Autodesk Fusion 360 part; units mm, degrees
(part 2 of 2)
sketch "Sketch6" plane through (0, 0, 2) normal (0, 0, 1) x (-1, 0, 0)
  spline S0 degree 3 poles (34.098, 26.8331) (34.098, 26.5964) (33.9796, 26.4781) (33.743, 26.4781) knots 0 0 0 0 1 1 1 1
  spline S1 degree 3 poles (33.743, 26.4781) (33.6225, 26.4812) (33.5343, 26.5113) (33.4772, 26.5694) knots 0 0 0 0 1 1 1 1
  spline S2 degree 3 poles (33.4772, 26.5694) (33.4206, 26.6276) (33.1512, 26.8965) (32.6695, 27.375) knots 0 0 0 0 1 1 1 1
  spline S3 degree 3 poles (32.6695, 27.375) (32.1935, 26.8991) (31.9257, 26.6307) (31.866, 26.5694) knots 0 0 0 0 1 1 1 1
  spline S4 degree 3 poles (31.866, 26.5694) (31.8068, 26.5087) (31.7181, 26.4781) (31.6003, 26.4781) knots 0 0 0 0 1 1 1 1
  spline S5 degree 3 poles (31.6003, 26.4781) (31.3636, 26.4796) (31.2447, 26.598) (31.2431, 26.8331) knots 0 0 0 0 1 1 1 1
  line L0 (31.2431, 26.8331) -> (31.2411, 28.9738)
  spline S6 degree 3 poles (31.2411, 28.9738) (31.2411, 29.2105) (31.3615, 29.3309) (31.6023, 29.335) knots 0 0 0 0 1 1 1 1
  spline S7 degree 3 poles (31.6023, 29.335) (31.838, 29.3335) (31.9569, 29.2136) (31.9594, 28.9738) knots 0 0 0 0 1 1 1 1
  line L1 (31.9594, 28.9738) -> (31.9594, 27.7135)
  spline S8 degree 3 poles (31.9594, 27.7135) (32.1993, 27.9585) (32.3487, 28.1116) (32.4079, 28.1723) knots 0 0 0 0 1 1 1 1
  spline S9 degree 3 poles (32.4079, 28.1723) (32.4661, 28.232) (32.5543, 28.2616) (32.6716, 28.2616) knots 0 0 0 0 1 1 1 1
  spline S10 degree 3 poles (32.6716, 28.2616) (32.7868, 28.2616) (32.8746, 28.2315) (32.9353, 28.1702) knots 0 0 0 0 1 1 1 1
  spline S11 degree 3 poles (32.9353, 28.1702) (32.9965, 28.108) (33.146, 27.9579) (33.3838, 27.7197) knots 0 0 0 0 1 1 1 1
  line L2 (33.3838, 27.7197) -> (33.3838, 28.9738)
  spline S12 degree 3 poles (33.3838, 28.9738) (33.3853, 29.2094) (33.5042, 29.3283) (33.7409, 29.3309) knots 0 0 0 0 1 1 1 1
  spline S13 degree 3 poles (33.7409, 29.3309) (33.9807, 29.3319) (34.0996, 29.2136) (34.098, 28.9738) knots 0 0 0 0 1 1 1 1
  line L3 (34.098, 28.9738) -> (34.098, 26.8331)
  spline S14 degree 3 poles (1.992, 26.8352) (1.992, 26.6001) (1.8731, 26.4812) (1.6349, 26.4781) knots 0 0 0 0 1 1 1 1
  line L4 (1.6349, 26.4781) -> (0.3871, 26.4781)
  spline S15 degree 3 poles (0.3871, 26.4781) (0.1504, 26.4781) (-0.0578, 26.5674) (-0.2379, 26.7459) knots 0 0 0 0 1 1 1 1
  spline S16 degree 3 poles (-0.2379, 26.7459) (-0.4191, 26.9245) (-0.5083, 27.1332) (-0.5057, 27.3709) knots 0 0 0 0 1 1 1 1
  spline S17 degree 3 poles (-0.5057, 27.3709) (-0.5026, 27.6091) (-0.4414, 27.7856) (-0.3209, 27.9003) knots 0 0 0 0 1 1 1 1
  spline S18 degree 3 poles (-0.3209, 27.9003) (-0.4466, 28.0239) (-0.5083, 28.2029) (-0.5057, 28.4381) knots 0 0 0 0 1 1 1 1
  spline S19 degree 3 poles (-0.5057, 28.4381) (-0.5042, 28.6737) (-0.4144, 28.8814) (-0.2358, 29.061) knots 0 0 0 0 1 1 1 1
  spline S20 degree 3 poles (-0.2358, 29.061) (-0.0573, 29.2411) (0.1431, 29.3309) (0.3642, 29.3309) knots 0 0 0 0 1 1 1 1
  line L5 (0.3642, 29.3309) -> (1.639, 29.3309)
  spline S21 degree 3 poles (1.639, 29.3309) (1.8747, 29.3335) (1.992, 29.2146) (1.992, 28.9738) knots 0 0 0 0 1 1 1 1
  line L6 (1.992, 28.9738) -> (1.992, 26.8352)
  spline S22 degree 3 poles (-8.0953, 26.5611) (-8.1587, 26.5004) (-8.249, 26.4698) (-8.3653, 26.4698) knots 0 0 0 0 1 1 1 1
  spline S23 degree 3 poles (-8.3653, 26.4698) (-8.4841, 26.4698) (-8.5734, 26.4999) (-8.6331, 26.5591) knots 0 0 0 0 1 1 1 1
  spline S24 degree 3 poles (-8.6331, 26.5591) (-8.6923, 26.6172) (-8.904, 26.8658) (-9.2684, 27.3044) knots 0 0 0 0 1 1 1 1
  spline S25 degree 3 poles (-9.2684, 27.3044) (-9.6364, 26.8575) (-9.8503, 26.6058) (-9.91, 26.5487) knots 0 0 0 0 1 1 1 1
  spline S26 degree 3 poles (-9.91, 26.5487) (-9.9707, 26.4905) (-10.0605, 26.4615) (-10.1799, 26.4615) knots 0 0 0 0 1 1 1 1
  spline S27 degree 3 poles (-10.1799, 26.4615) (-10.2962, 26.4615) (-10.3855, 26.4921) (-10.4477, 26.5528) knots 0 0 0 0 1 1 1 1
  spline S28 degree 3 poles (-10.4477, 26.5528) (-10.51, 26.6125) (-10.5396, 26.7023) (-10.537, 26.8227) knots 0 0 0 0 1 1 1 1
  spline S29 degree 3 poles (-10.537, 26.8227) (-10.537, 26.9489) (-10.4737, 27.0667) (-10.3481, 27.1757) knots 0 0 0 0 1 1 1 1
  line L7 (-10.3481, 27.1757) -> (-9.7397, 27.892)
  line L8 (-9.7397, 27.892) -> (-10.3481, 28.6021)
  spline S30 degree 3 poles (-10.3481, 28.6021) (-10.482, 28.7282) (-10.5443, 28.8492) (-10.5349, 28.9655) knots 0 0 0 0 1 1 1 1
  spline S31 degree 3 poles (-10.5349, 28.9655) (-10.5401, 29.0859) (-10.5105, 29.1762) (-10.4457, 29.2354) knots 0 0 0 0 1 1 1 1
  spline S32 degree 3 poles (-10.4457, 29.2354) (-10.3803, 29.2951) (-10.2905, 29.3241) (-10.1758, 29.3226) knots 0 0 0 0 1 1 1 1
  spline S33 degree 3 poles (-10.1758, 29.3226) (-10.0522, 29.3241) (-9.9603, 29.293) (-9.8996, 29.2291) knots 0 0 0 0 1 1 1 1
  spline S34 degree 3 poles (-9.8996, 29.2291) (-9.8384, 29.1658) (-9.6307, 28.9193) (-9.2767, 28.49) knots 0 0 0 0 1 1 1 1
  spline S35 degree 3 poles (-9.2767, 28.49) (-8.9155, 28.9276) (-8.7042, 29.1772) (-8.6435, 29.2395) knots 0 0 0 0 1 1 1 1
  spline S36 degree 3 poles (-8.6435, 29.2395) (-8.5822, 29.3018) (-8.4903, 29.3319) (-8.3673, 29.3309) knots 0 0 0 0 1 1 1 1
  spline S37 degree 3 poles (-8.3673, 29.3309) (-8.2521, 29.3335) (-8.1623, 29.3054) (-8.0974, 29.2457) knots 0 0 0 0 1 1 1 1
  spline S38 degree 3 poles (-8.0974, 29.2457) (-8.032, 29.185) (-8.0029, 29.0942) (-8.0102, 28.9738) knots 0 0 0 0 1 1 1 1
  spline S39 degree 3 poles (-8.0102, 28.9738) (-7.9988, 28.8575) (-8.0606, 28.7371) (-8.195, 28.6125) knots 0 0 0 0 1 1 1 1
  line L9 (-8.195, 28.6125) -> (-8.8303, 27.9024)
  line L10 (-8.8303, 27.9024) -> (-8.1971, 27.1861)
  spline S40 degree 3 poles (-8.1971, 27.1861) (-8.0709, 27.0755) (-8.0081, 26.9572) (-8.0081, 26.8311) knots 0 0 0 0 1 1 1 1
  spline S41 degree 3 poles (-8.0081, 26.8311) (-8.004, 26.7106) (-8.033, 26.6208) (-8.0953, 26.5611) knots 0 0 0 0 1 1 1 1
  spline S42 degree 3 poles (13.2978, 6.9999) (13.8352, 7.003) (14.106, 6.7343) (14.1081, 6.1938) knots 0 0 0 0 1 1 1 1
  spline S43 degree 3 poles (14.1081, 6.1938) (14.1029, 5.6543) (13.8342, 5.3794) (13.3019, 5.3711) knots 0 0 0 0 1 1 1 1
  line L11 (13.3019, 5.3711) -> (11.6648, 5.3711)
  spline S44 degree 3 poles (11.6648, 5.3711) (11.1222, 5.3773) (10.8463, 5.6481) (10.838, 6.1855) knots 0 0 0 0 1 1 1 1
  spline S45 degree 3 poles (10.838, 6.1855) (10.8494, 6.7292) (11.1233, 6.9999) (11.6607, 6.9999) knots 0 0 0 0 1 1 1 1
  line L12 (11.6607, 6.9999) -> (13.2978, 6.9999)
  spline S46 degree 3 poles (24.2533, 2.9237) (23.7158, 2.9268) (23.4451, 3.1986) (23.4388, 3.7381) knots 0 0 0 0 1 1 1 1
  spline S47 degree 3 poles (23.4388, 3.7381) (23.4388, 4.2818) (23.7014, 4.5546) (24.2243, 4.5567) knots 0 0 0 0 1 1 1 1
  line L13 (24.2243, 4.5567) -> (26.7007, 4.5525)
  spline S48 degree 3 poles (26.7007, 4.5525) (27.2495, 4.5587) (27.5265, 4.6962) (27.5316, 4.966) knots 0 0 0 0 1 1 1 1
  spline S49 degree 3 poles (27.5316, 4.966) (27.5234, 5.2254) (27.2453, 5.3535) (26.6965, 5.3504) knots 0 0 0 0 1 1 1 1
  line L14 (26.6965, 5.3504) -> (25.8945, 5.3504)
  spline S50 degree 3 poles (25.8945, 5.3504) (24.2605, 5.3566) (23.4388, 6.0439) (23.4306, 7.4134) knots 0 0 0 0 1 1 1 1
  spline S51 degree 3 poles (23.4306, 7.4134) (23.4306, 8.7445) (24.2512, 9.4143) (25.8904, 9.4225) knots 0 0 0 0 1 1 1 1
  line L15 (25.8904, 9.4225) -> (28.3378, 9.4225)
  spline S52 degree 3 poles (28.3378, 9.4225) (28.8814, 9.4205) (29.1512, 9.1538) (29.1481, 8.6247) knots 0 0 0 0 1 1 1 1
  spline S53 degree 3 poles (29.1481, 8.6247) (29.146, 8.0851) (28.8783, 7.8175) (28.346, 7.8226) knots 0 0 0 0 1 1 1 1
  line L16 (28.346, 7.8226) -> (25.8904, 7.8102)
  spline S54 degree 3 poles (25.8904, 7.8102) (25.3447, 7.8082) (25.0718, 7.6686) (25.0718, 7.3927) knots 0 0 0 0 1 1 1 1
  spline S55 degree 3 poles (25.0718, 7.3927) (25.0718, 7.1147) (25.3478, 6.9772) (25.8986, 6.9793) knots 0 0 0 0 1 1 1 1
  line L17 (25.8986, 6.9793) -> (26.7007, 6.9793)
  spline S56 degree 3 poles (26.7007, 6.9793) (28.3326, 6.9772) (29.1481, 6.3054) (29.1481, 4.966) knots 0 0 0 0 1 1 1 1
  spline S57 degree 3 poles (29.1481, 4.966) (29.1594, 3.6079) (28.344, 2.9268) (26.7007, 2.9237) knots 0 0 0 0 1 1 1 1
  line L18 (26.7007, 2.9237) -> (24.2533, 2.9237)
  spline S58 degree 3 poles (16.1297, 3.7381) (16.1276, 3.2007) (15.8558, 2.9268) (15.3153, 2.9154) knots 0 0 0 0 1 1 1 1
  line L19 (15.3153, 2.9154) -> (11.1977, 2.9237)
  spline S59 degree 3 poles (11.1977, 2.9237) (10.6912, 2.932) (10.436, 3.1955) (10.4329, 3.7133) knots 0 0 0 0 1 1 1 1
  spline S60 degree 3 poles (10.4329, 3.7133) (10.4329, 4.2673) (10.7078, 4.5484) (11.2556, 4.5567) knots 0 0 0 0 1 1 1 1
  line L20 (11.2556, 4.5567) -> (14.4967, 4.5567)
  line L21 (14.4967, 4.5567) -> (14.4967, 7.7978)
  line L22 (14.4967, 7.7978) -> (11.2638, 7.7978)
  spline S61 degree 3 poles (11.2638, 7.7978) (10.716, 7.8009) (10.4411, 8.0748) (10.4411, 8.6205) knots 0 0 0 0 1 1 1 1
  spline S62 degree 3 poles (10.4411, 8.6205) (10.4442, 9.1559) (10.7129, 9.4256) (11.2473, 9.4308) knots 0 0 0 0 1 1 1 1
  line L23 (11.2473, 9.4308) -> (15.3153, 9.4308)
  spline S63 degree 3 poles (15.3153, 9.4308) (15.8558, 9.4308) (16.1276, 9.1683) (16.1297, 8.6412) knots 0 0 0 0 1 1 1 1
  line L24 (16.1297, 8.6412) -> (16.1297, 3.7381)
  spline S64 degree 3 poles (-1.5825, 26.6629) (-1.8109, 26.5399) (-2.046, 26.4781) (-2.2884, 26.4781) knots 0 0 0 0 1 1 1 1
  spline S65 degree 3 poles (-2.2884, 26.4781) (-2.5277, 26.4781) (-2.7608, 26.5399) (-2.9881, 26.6629) knots 0 0 0 0 1 1 1 1
  spline S66 degree 3 poles (-2.9881, 26.6629) (-3.2165, 26.7864) (-3.3951, 26.9629) (-3.5238, 27.1923) knots 0 0 0 0 1 1 1 1
  spline S67 degree 3 poles (-3.5238, 27.1923) (-3.6536, 27.4207) (-3.719, 27.659) (-3.719, 27.9066) knots 0 0 0 0 1 1 1 1
  spline S68 degree 3 poles (-3.719, 27.9066) (-3.719, 28.1547) (-3.6557, 28.3919) (-3.53, 28.6187) knots 0 0 0 0 1 1 1 1
  spline S69 degree 3 poles (-3.53, 28.6187) (-3.4055, 28.8445) (-3.229, 29.0205) (-3.0006, 29.1461) knots 0 0 0 0 1 1 1 1
  spline S70 degree 3 poles (-3.0006, 29.1461) (-2.7732, 29.2722) (-2.536, 29.335) (-2.2884, 29.335) knots 0 0 0 0 1 1 1 1
  spline S71 degree 3 poles (-2.2884, 29.335) (-2.0419, 29.335) (-1.8047, 29.2722) (-1.5763, 29.1461) knots 0 0 0 0 1 1 1 1
  spline S72 degree 3 poles (-1.5763, 29.1461) (-1.3489, 29.0205) (-1.1724, 28.8445) (-1.0468, 28.6187) knots 0 0 0 0 1 1 1 1
  spline S73 degree 3 poles (-1.0468, 28.6187) (-0.9223, 28.3919) (-0.86, 28.1547) (-0.86, 27.9066) knots 0 0 0 0 1 1 1 1
  spline S74 degree 3 poles (-0.86, 27.9066) (-0.86, 27.659) (-0.9233, 27.4207) (-1.051, 27.1923) knots 0 0 0 0 1 1 1 1
  spline S75 degree 3 poles (-1.051, 27.1923) (-1.1782, 26.9629) (-1.3552, 26.7864) (-1.5825, 26.6629) knots 0 0 0 0 1 1 1 1
  spline S76 degree 3 poles (9.664, 28.2658) (9.8996, 28.2673) (10.018, 28.1495) (10.019, 27.9128) knots 0 0 0 0 1 1 1 1
  spline S77 degree 3 poles (10.019, 27.9128) (10.0164, 27.6751) (9.8986, 27.5536) (9.666, 27.5494) knots 0 0 0 0 1 1 1 1
  line L25 (9.666, 27.5494) -> (8.9476, 27.5494)
  spline S78 degree 3 poles (8.9476, 27.5494) (8.7099, 27.5526) (8.5895, 27.6719) (8.5864, 27.9086) knots 0 0 0 0 1 1 1 1
  spline S79 degree 3 poles (8.5864, 27.9086) (8.5905, 28.1469) (8.7104, 28.2658) (8.9456, 28.2658) knots 0 0 0 0 1 1 1 1
  line L26 (8.9456, 28.2658) -> (9.664, 28.2658)
  spline S80 degree 3 poles (21.9665, 26.8311) (21.9655, 26.5985) (21.8461, 26.4812) (21.6094, 26.4781) knots 0 0 0 0 1 1 1 1
  line L27 (21.6094, 26.4781) -> (20.3574, 26.4781)
  spline S81 degree 3 poles (20.3574, 26.4781) (20.1238, 26.4781) (19.9172, 26.5684) (19.7387, 26.748) knots 0 0 0 0 1 1 1 1
  spline S82 degree 3 poles (19.7387, 26.748) (19.5591, 26.9281) (19.4698, 27.1342) (19.4708, 27.3667) knots 0 0 0 0 1 1 1 1
  spline S83 degree 3 poles (19.4708, 27.3667) (19.4708, 27.6133) (19.516, 27.8214) (19.6058, 27.9917) knots 0 0 0 0 1 1 1 1
  spline S84 degree 3 poles (19.6058, 27.9917) (19.6945, 28.1609) (19.8295, 28.2481) (20.0107, 28.2533) knots 0 0 0 0 1 1 1 1
  line L28 (20.0107, 28.2533) -> (19.5705, 28.6997)
  spline S85 degree 3 poles (19.5705, 28.6997) (19.4999, 28.7692) (19.4646, 28.8611) (19.4646, 28.9758) knots 0 0 0 0 1 1 1 1
  spline S86 degree 3 poles (19.4646, 28.9758) (19.4688, 29.2141) (19.5881, 29.3319) (19.8217, 29.3309) knots 0 0 0 0 1 1 1 1
  spline S87 degree 3 poles (19.8217, 29.3309) (19.9437, 29.335) (20.0636, 29.2769) (20.1809, 29.1565) knots 0 0 0 0 1 1 1 1
  line L29 (20.1809, 29.1565) -> (20.8951, 28.272)
  spline S88 degree 3 poles (20.8951, 28.272) (21.0145, 28.1448) (21.0747, 28.0218) (21.0758, 27.9024) knots 0 0 0 0 1 1 1 1
  spline S89 degree 3 poles (21.0758, 27.9024) (21.0758, 27.6631) (20.9564, 27.5443) (20.7166, 27.5453) knots 0 0 0 0 1 1 1 1
  line L30 (20.7166, 27.5453) -> (20.4633, 27.5432)
  spline S90 degree 3 poles (20.4633, 27.5432) (20.2754, 27.5463) (20.182, 27.4887) (20.183, 27.3709) knots 0 0 0 0 1 1 1 1
  spline S91 degree 3 poles (20.183, 27.3709) (20.183, 27.252) (20.2764, 27.1923) (20.4633, 27.1923) knots 0 0 0 0 1 1 1 1
  line L31 (20.4633, 27.1923) -> (21.2502, 27.1923)
  line L32 (21.2502, 27.1923) -> (21.2502, 28.9738)
  spline S92 degree 3 poles (21.2502, 28.9738) (21.2502, 29.212) (21.3701, 29.3309) (21.6094, 29.3309) knots 0 0 0 0 1 1 1 1
  spline S93 degree 3 poles (21.6094, 29.3309) (21.8492, 29.3319) (21.9681, 29.2146) (21.9665, 28.9779) knots 0 0 0 0 1 1 1 1
  line L33 (21.9665, 28.9779) -> (21.9665, 26.8311)
  spline S94 degree 3 poles (30.8875, 26.8352) (30.8864, 26.6001) (30.7671, 26.4796) (30.5304, 26.4739) knots 0 0 0 0 1 1 1 1
  line L34 (30.5304, 26.4739) -> (28.724, 26.4781)
  spline S95 degree 3 poles (28.724, 26.4781) (28.5029, 26.4812) (28.3913, 26.5964) (28.3897, 26.8248) knots 0 0 0 0 1 1 1 1
  spline S96 degree 3 poles (28.3897, 26.8248) (28.3897, 27.0672) (28.5096, 27.1897) (28.7489, 27.1923) knots 0 0 0 0 1 1 1 1
  line L35 (28.7489, 27.1923) -> (30.1712, 27.1923)
  line L36 (30.1712, 27.1923) -> (30.1712, 28.6146)
  line L37 (30.1712, 28.6146) -> (28.7531, 28.6146)
  spline S97 degree 3 poles (28.7531, 28.6146) (28.5138, 28.6161) (28.3939, 28.7365) (28.3939, 28.9758) knots 0 0 0 0 1 1 1 1
  spline S98 degree 3 poles (28.3939, 28.9758) (28.3939, 29.2099) (28.5117, 29.3283) (28.7469, 29.3309) knots 0 0 0 0 1 1 1 1
  line L38 (28.7469, 29.3309) -> (30.5304, 29.3309)
  spline S99 degree 3 poles (30.5304, 29.3309) (30.7671, 29.3309) (30.8864, 29.2156) (30.8875, 28.9841) knots 0 0 0 0 1 1 1 1
  line L39 (30.8875, 28.9841) -> (30.8875, 26.8352)
  spline S100 degree 3 poles (28.0331, 26.8331) (28.0331, 26.5964) (27.9148, 26.4781) (27.6781, 26.4781) knots 0 0 0 0 1 1 1 1
  spline S101 degree 3 poles (27.6781, 26.4781) (27.5577, 26.4812) (27.4694, 26.5113) (27.4123, 26.5694) knots 0 0 0 0 1 1 1 1
  spline S102 degree 3 poles (27.4123, 26.5694) (27.3558, 26.6276) (27.0864, 26.8965) (26.6047, 27.375) knots 0 0 0 0 1 1 1 1
  spline S103 degree 3 poles (26.6047, 27.375) (26.1287, 26.8991) (25.8608, 26.6307) (25.8012, 26.5694) knots 0 0 0 0 1 1 1 1
  spline S104 degree 3 poles (25.8012, 26.5694) (25.742, 26.5087) (25.6532, 26.4781) (25.5354, 26.4781) knots 0 0 0 0 1 1 1 1
  spline S105 degree 3 poles (25.5354, 26.4781) (25.2987, 26.4796) (25.1798, 26.598) (25.1783, 26.8331) knots 0 0 0 0 1 1 1 1
  line L40 (25.1783, 26.8331) -> (25.1762, 28.9738)
  spline S106 degree 3 poles (25.1762, 28.9738) (25.1762, 29.2105) (25.2966, 29.3309) (25.5375, 29.335) knots 0 0 0 0 1 1 1 1
  spline S107 degree 3 poles (25.5375, 29.335) (25.7731, 29.3335) (25.892, 29.2136) (25.8946, 28.9738) knots 0 0 0 0 1 1 1 1
  line L41 (25.8946, 28.9738) -> (25.8946, 27.7135)
  spline S108 degree 3 poles (25.8946, 27.7135) (26.1344, 27.9585) (26.2839, 28.1116) (26.3431, 28.1723) knots 0 0 0 0 1 1 1 1
  spline S109 degree 3 poles (26.3431, 28.1723) (26.4012, 28.232) (26.4894, 28.2616) (26.6067, 28.2616) knots 0 0 0 0 1 1 1 1
  spline S110 degree 3 poles (26.6067, 28.2616) (26.722, 28.2616) (26.8097, 28.2315) (26.8704, 28.1702) knots 0 0 0 0 1 1 1 1
  spline S111 degree 3 poles (26.8704, 28.1702) (26.9317, 28.108) (27.0812, 27.9579) (27.3189, 27.7197) knots 0 0 0 0 1 1 1 1
  line L42 (27.3189, 27.7197) -> (27.3189, 28.9738)
  spline S112 degree 3 poles (27.3189, 28.9738) (27.3205, 29.2094) (27.4393, 29.3283) (27.676, 29.3309) knots 0 0 0 0 1 1 1 1
  spline S113 degree 3 poles (27.676, 29.3309) (27.9158, 29.3319) (28.0347, 29.2136) (28.0331, 28.9738) knots 0 0 0 0 1 1 1 1
  line L43 (28.0331, 28.9738) -> (28.0331, 26.8331)
  spline S114 degree 3 poles (14.1161, 26.8331) (14.1161, 26.5964) (13.9977, 26.4781) (13.761, 26.4781) knots 0 0 0 0 1 1 1 1
  spline S115 degree 3 poles (13.761, 26.4781) (13.6406, 26.4812) (13.5524, 26.5113) (13.4953, 26.5694) knots 0 0 0 0 1 1 1 1
  spline S116 degree 3 poles (13.4953, 26.5694) (13.4387, 26.6276) (13.1693, 26.8965) (12.6876, 27.375) knots 0 0 0 0 1 1 1 1
  spline S117 degree 3 poles (12.6876, 27.375) (12.2116, 26.8991) (11.9438, 26.6307) (11.8841, 26.5694) knots 0 0 0 0 1 1 1 1
  spline S118 degree 3 poles (11.8841, 26.5694) (11.8249, 26.5087) (11.7362, 26.4781) (11.6183, 26.4781) knots 0 0 0 0 1 1 1 1
  spline S119 degree 3 poles (11.6183, 26.4781) (11.3816, 26.4796) (11.2628, 26.598) (11.2612, 26.8331) knots 0 0 0 0 1 1 1 1
  line L44 (11.2612, 26.8331) -> (11.2591, 28.9738)
  spline S120 degree 3 poles (11.2591, 28.9738) (11.2591, 29.2105) (11.3796, 29.3309) (11.6204, 29.335) knots 0 0 0 0 1 1 1 1
  spline S121 degree 3 poles (11.6204, 29.335) (11.8561, 29.3335) (11.9749, 29.2136) (11.9775, 28.9738) knots 0 0 0 0 1 1 1 1
  line L45 (11.9775, 28.9738) -> (11.9775, 27.7135)
  spline S122 degree 3 poles (11.9775, 27.7135) (12.2173, 27.9585) (12.3668, 28.1116) (12.426, 28.1723) knots 0 0 0 0 1 1 1 1
  spline S123 degree 3 poles (12.426, 28.1723) (12.4841, 28.232) (12.5724, 28.2616) (12.6897, 28.2616) knots 0 0 0 0 1 1 1 1
  spline S124 degree 3 poles (12.6897, 28.2616) (12.8049, 28.2616) (12.8926, 28.2315) (12.9534, 28.1702) knots 0 0 0 0 1 1 1 1
  spline S125 degree 3 poles (12.9534, 28.1702) (13.0146, 28.108) (13.1641, 27.9579) (13.4018, 27.7197) knots 0 0 0 0 1 1 1 1
  line L46 (13.4018, 27.7197) -> (13.4018, 28.9738)
  spline S126 degree 3 poles (13.4018, 28.9738) (13.4034, 29.2094) (13.5223, 29.3283) (13.759, 29.3309) knots 0 0 0 0 1 1 1 1
  spline S127 degree 3 poles (13.759, 29.3309) (13.9988, 29.3319) (14.1176, 29.2136) (14.1161, 28.9738) knots 0 0 0 0 1 1 1 1
  line L47 (14.1161, 28.9738) -> (14.1161, 26.8331)
  spline S128 degree 3 poles (18.3923, 26.6629) (18.1639, 26.5399) (17.9288, 26.4781) (17.6863, 26.4781) knots 0 0 0 0 1 1 1 1
  spline S129 degree 3 poles (17.6863, 26.4781) (17.4471, 26.4781) (17.214, 26.5399) (16.9866, 26.6629) knots 0 0 0 0 1 1 1 1
  spline S130 degree 3 poles (16.9866, 26.6629) (16.7583, 26.7864) (16.5797, 26.9629) (16.451, 27.1923) knots 0 0 0 0 1 1 1 1
  spline S131 degree 3 poles (16.451, 27.1923) (16.3212, 27.4207) (16.2558, 27.659) (16.2558, 27.9066) knots 0 0 0 0 1 1 1 1
  spline S132 degree 3 poles (16.2558, 27.9066) (16.2558, 28.1547) (16.3191, 28.3919) (16.4447, 28.6187) knots 0 0 0 0 1 1 1 1
  spline S133 degree 3 poles (16.4447, 28.6187) (16.5693, 28.8445) (16.7458, 29.0205) (16.9742, 29.1461) knots 0 0 0 0 1 1 1 1
  spline S134 degree 3 poles (16.9742, 29.1461) (17.2015, 29.2722) (17.4388, 29.335) (17.6863, 29.335) knots 0 0 0 0 1 1 1 1
  spline S135 degree 3 poles (17.6863, 29.335) (17.9329, 29.335) (18.1701, 29.2722) (18.3985, 29.1461) knots 0 0 0 0 1 1 1 1
  spline S136 degree 3 poles (18.3985, 29.1461) (18.6259, 29.0205) (18.8023, 28.8445) (18.928, 28.6187) knots 0 0 0 0 1 1 1 1
  spline S137 degree 3 poles (18.928, 28.6187) (19.0525, 28.3919) (19.1148, 28.1547) (19.1148, 27.9066) knots 0 0 0 0 1 1 1 1
  spline S138 degree 3 poles (19.1148, 27.9066) (19.1148, 27.659) (19.0515, 27.4207) (18.9238, 27.1923) knots 0 0 0 0 1 1 1 1
  spline S139 degree 3 poles (18.9238, 27.1923) (18.7966, 26.9629) (18.6196, 26.7864) (18.3923, 26.6629) knots 0 0 0 0 1 1 1 1
  spline S140 degree 3 poles (29.6459, 28.2658) (29.8815, 28.2673) (29.9999, 28.1495) (30.0009, 27.9128) knots 0 0 0 0 1 1 1 1
  spline S141 degree 3 poles (30.0009, 27.9128) (29.9983, 27.6751) (29.8805, 27.5536) (29.648, 27.5494) knots 0 0 0 0 1 1 1 1
  line L48 (29.648, 27.5494) -> (28.9296, 27.5494)
  spline S142 degree 3 poles (28.9296, 27.5494) (28.6918, 27.5526) (28.5714, 27.6719) (28.5683, 27.9086) knots 0 0 0 0 1 1 1 1
  spline S143 degree 3 poles (28.5683, 27.9086) (28.5724, 28.1469) (28.6924, 28.2658) (28.9275, 28.2658) knots 0 0 0 0 1 1 1 1
  line L49 (28.9275, 28.2658) -> (29.6459, 28.2658)
  line L50 (7, -12) -> (17, -12)
  line L51 (17, -12) -> (17, -15)
  line L52 (17, -15) -> (7, -15)
  line L53 (7, -15) -> (7, -12)
  arc A0 (37, 80) -> (35, 82) centre (35, 80) ccw
  line L54 (35, 82) -> (-11, 82)
  arc A1 (-11, 82) -> (-13, 80) centre (-11, 80) ccw
  line L55 (-13, 80) -> (-13, -16)
  arc A2 (-13, -16) -> (-11, -18) centre (-11, -16) ccw
  line L56 (-11, -18) -> (35, -18)
  arc A3 (35, -18) -> (37, -16) centre (35, -16) ccw
  line L57 (37, -16) -> (37, 80)
  spline S144 degree 3 poles (8.0533, 26.8352) (8.0523, 26.6001) (7.9329, 26.4796) (7.6962, 26.4739) knots 0 0 0 0 1 1 1 1
  line L58 (7.6962, 26.4739) -> (5.8898, 26.4781)
  spline S145 degree 3 poles (5.8898, 26.4781) (5.6687, 26.4812) (5.5571, 26.5964) (5.5556, 26.8248) knots 0 0 0 0 1 1 1 1
  spline S146 degree 3 poles (5.5556, 26.8248) (5.5556, 27.0672) (5.6755, 27.1897) (5.9147, 27.1923) knots 0 0 0 0 1 1 1 1
  line L59 (5.9147, 27.1923) -> (6.4483, 27.1923)
  line L60 (6.4483, 27.1923) -> (6.4483, 28.9758)
  spline S147 degree 3 poles (6.4483, 28.9758) (6.4499, 29.2099) (6.5688, 29.3283) (6.8055, 29.3309) knots 0 0 0 0 1 1 1 1
  spline S148 degree 3 poles (6.8055, 29.3309) (7.0437, 29.3309) (7.1626, 29.2156) (7.1626, 28.9841) knots 0 0 0 0 1 1 1 1
  line L61 (7.1626, 28.9841) -> (7.1605, 27.1923)
  line L62 (7.1605, 27.1923) -> (7.6962, 27.1923)
  spline S149 degree 3 poles (7.6962, 27.1923) (7.9344, 27.1923) (8.0533, 27.0735) (8.0533, 26.8352) knots 0 0 0 0 1 1 1 1
  spline S150 degree 3 poles (-4.0746, 26.8352) (-4.0757, 26.6001) (-4.1951, 26.4796) (-4.4317, 26.4739) knots 0 0 0 0 1 1 1 1
  line L63 (-4.4317, 26.4739) -> (-6.2381, 26.4781)
  spline S151 degree 3 poles (-6.2381, 26.4781) (-6.4592, 26.4812) (-6.5708, 26.5964) (-6.5724, 26.8248) knots 0 0 0 0 1 1 1 1
  spline S152 degree 3 poles (-6.5724, 26.8248) (-6.5724, 27.0672) (-6.4525, 27.1897) (-6.2132, 27.1923) knots 0 0 0 0 1 1 1 1
  line L64 (-6.2132, 27.1923) -> (-5.6796, 27.1923)
  line L65 (-5.6796, 27.1923) -> (-5.6796, 28.9758)
  spline S153 degree 3 poles (-5.6796, 28.9758) (-5.678, 29.2099) (-5.5592, 29.3283) (-5.3225, 29.3309) knots 0 0 0 0 1 1 1 1
  spline S154 degree 3 poles (-5.3225, 29.3309) (-5.0842, 29.3309) (-4.9653, 29.2156) (-4.9653, 28.9841) knots 0 0 0 0 1 1 1 1
  line L66 (-4.9653, 28.9841) -> (-4.9674, 27.1923)
  line L67 (-4.9674, 27.1923) -> (-4.4317, 27.1923)
  spline S155 degree 3 poles (-4.4317, 27.1923) (-4.1935, 27.1923) (-4.0746, 27.0735) (-4.0746, 26.8352) knots 0 0 0 0 1 1 1 1
  spline S156 degree 3 poles (5.5489, 3.7299) (5.5468, 3.1986) (5.275, 2.9299) (4.7344, 2.9237) knots 0 0 0 0 1 1 1 1
  line L68 (4.7344, 2.9237) -> (1.8778, 2.9237)
  spline S157 degree 3 poles (1.8778, 2.9237) (1.3465, 2.9237) (0.8763, 3.1294) (0.468, 3.5397) knots 0 0 0 0 1 1 1 1
  spline S158 degree 3 poles (0.468, 3.5397) (0.0577, 3.951) (-0.1459, 4.4203) (-0.1438, 4.9494) knots 0 0 0 0 1 1 1 1
  spline S159 degree 3 poles (-0.1438, 4.9494) (-0.1438, 5.5117) (-0.0415, 5.9871) (0.1621, 6.3757) knots 0 0 0 0 1 1 1 1
  spline S160 degree 3 poles (0.1621, 6.3757) (0.3667, 6.7622) (0.6747, 6.9607) (1.0881, 6.971) knots 0 0 0 0 1 1 1 1
  line L69 (1.0881, 6.971) -> (0.0836, 7.9921)
  spline S161 degree 3 poles (0.0836, 7.9921) (-0.0756, 8.1523) (-0.1562, 8.3621) (-0.1562, 8.6205) knots 0 0 0 0 1 1 1 1
  spline S162 degree 3 poles (-0.1562, 8.6205) (-0.148, 9.1642) (0.1239, 9.4329) (0.6582, 9.4308) knots 0 0 0 0 1 1 1 1
  spline S163 degree 3 poles (0.6582, 9.4308) (0.9342, 9.4391) (1.207, 9.3068) (1.4768, 9.0339) knots 0 0 0 0 1 1 1 1
  line L70 (1.4768, 9.0339) -> (3.1015, 7.0123)
  spline S164 degree 3 poles (3.1015, 7.0123) (3.3774, 6.723) (3.5169, 6.4439) (3.519, 6.1731) knots 0 0 0 0 1 1 1 1
  spline S165 degree 3 poles (3.519, 6.1731) (3.519, 5.6274) (3.2451, 5.3566) (2.6963, 5.3587) knots 0 0 0 0 1 1 1 1
  line L71 (2.6963, 5.3587) -> (2.1175, 5.3546)
  spline S166 degree 3 poles (2.1175, 5.3546) (1.6907, 5.3608) (1.4799, 5.2285) (1.485, 4.9577) knots 0 0 0 0 1 1 1 1
  spline S167 degree 3 poles (1.485, 4.9577) (1.485, 4.691) (1.6979, 4.5567) (2.1217, 4.5567) knots 0 0 0 0 1 1 1 1
  line L72 (2.1217, 4.5567) -> (3.9159, 4.5567)
  line L73 (3.9159, 4.5567) -> (3.9159, 8.6164)
  spline S168 degree 3 poles (3.9159, 8.6164) (3.9138, 9.16) (4.1867, 9.4308) (4.7344, 9.4308) knots 0 0 0 0 1 1 1 1
  spline S169 degree 3 poles (4.7344, 9.4308) (5.2801, 9.4329) (5.552, 9.1652) (5.5489, 8.6247) knots 0 0 0 0 1 1 1 1
  line L74 (5.5489, 8.6247) -> (5.5489, 3.7299)
  spline S170 degree 3 poles (18.577, 3.7299) (18.577, 3.1821) (18.3042, 2.9072) (17.7584, 2.9072) knots 0 0 0 0 1 1 1 1
  spline S171 degree 3 poles (17.7584, 2.9072) (17.2189, 2.9072) (16.9471, 3.1821) (16.944, 3.7299) knots 0 0 0 0 1 1 1 1
  line L75 (16.944, 3.7299) -> (16.9482, 8.6164)
  spline S172 degree 3 poles (16.9482, 8.6164) (16.9482, 9.1652) (17.221, 9.436) (17.7667, 9.4308) knots 0 0 0 0 1 1 1 1
  spline S173 degree 3 poles (17.7667, 9.4308) (18.3104, 9.4329) (18.5801, 9.1652) (18.577, 8.6247) knots 0 0 0 0 1 1 1 1
  line L76 (18.577, 8.6247) -> (18.577, 6.9834)
  line L77 (18.577, 6.9834) -> (19.7718, 6.9875)
  spline S174 degree 3 poles (19.7718, 6.9875) (20.3288, 6.9875) (20.611, 6.7178) (20.6193, 6.1773) knots 0 0 0 0 1 1 1 1
  spline S175 degree 3 poles (20.6193, 6.1773) (20.6172, 5.6347) (20.334, 5.3649) (19.7718, 5.367) knots 0 0 0 0 1 1 1 1
  line L78 (19.7718, 5.367) -> (18.577, 5.3546)
  line L79 (18.577, 5.3546) -> (18.577, 3.7299)
  spline S176 degree 3 poles (22.6408, 3.7381) (22.6408, 3.1955) (22.3701, 2.9216) (21.8264, 2.9154) knots 0 0 0 0 1 1 1 1
  spline S177 degree 3 poles (21.8264, 2.9154) (21.2807, 2.9185) (21.0079, 3.1914) (21.0079, 3.734) knots 0 0 0 0 1 1 1 1
  line L80 (21.0079, 3.734) -> (21.012, 8.6164)
  spline S178 degree 3 poles (21.012, 8.6164) (21.0151, 9.1538) (21.2879, 9.4256) (21.8306, 9.4308) knots 0 0 0 0 1 1 1 1
  spline S179 degree 3 poles (21.8306, 9.4308) (22.3742, 9.4287) (22.6439, 9.158) (22.6408, 8.6205) knots 0 0 0 0 1 1 1 1
  line L81 (22.6408, 8.6205) -> (22.6408, 3.7381)
  spline S180 degree 3 poles (8.804, 6.9999) (9.3414, 7.003) (9.6122, 6.7343) (9.6142, 6.1938) knots 0 0 0 0 1 1 1 1
  spline S181 degree 3 poles (9.6142, 6.1938) (9.6091, 5.6543) (9.3404, 5.3794) (8.8081, 5.3711) knots 0 0 0 0 1 1 1 1
  line L82 (8.8081, 5.3711) -> (7.171, 5.3711)
  spline S182 degree 3 poles (7.171, 5.3711) (6.6315, 5.3773) (6.3566, 5.6481) (6.3483, 6.1855) knots 0 0 0 0 1 1 1 1
  spline S183 degree 3 poles (6.3483, 6.1855) (6.3597, 6.7292) (6.6325, 6.9999) (7.1668, 6.9999) knots 0 0 0 0 1 1 1 1
  line L83 (7.1668, 6.9999) -> (8.804, 6.9999)
  spline S184 degree 3 poles (-6.929, 26.8331) (-6.9274, 26.598) (-7.0452, 26.4796) (-7.2819, 26.4781) knots 0 0 0 0 1 1 1 1
  spline S185 degree 3 poles (-7.2819, 26.4781) (-7.5197, 26.4812) (-7.6411, 26.5985) (-7.6453, 26.8311) knots 0 0 0 0 1 1 1 1
  line L84 (-7.6453, 26.8311) -> (-7.6453, 28.9758)
  spline S186 degree 3 poles (-7.6453, 28.9758) (-7.6422, 29.2141) (-7.5228, 29.334) (-7.2861, 29.3371) knots 0 0 0 0 1 1 1 1
  spline S187 degree 3 poles (-7.2861, 29.3371) (-7.0478, 29.333) (-6.929, 29.2136) (-6.929, 28.9779) knots 0 0 0 0 1 1 1 1
  line L85 (-6.929, 28.9779) -> (-6.929, 26.8331)
  line L86 (2.7033, 29.333) -> (4.8418, 29.333)
  spline S188 degree 3 poles (4.8418, 29.333) (4.9031, 29.333) (4.9617, 29.3179) (5.0183, 29.2873) knots 0 0 0 0 1 1 1 1
  spline S189 degree 3 poles (5.0183, 29.2873) (5.0754, 29.2572) (5.1195, 29.2136) (5.1512, 29.1565) knots 0 0 0 0 1 1 1 1
  spline S190 degree 3 poles (5.1512, 29.1565) (5.1834, 29.0999) (5.199, 29.0397) (5.199, 28.9758) knots 0 0 0 0 1 1 1 1
  spline S191 degree 3 poles (5.199, 28.9758) (5.199, 28.9135) (5.0214, 28.5253) (4.6654, 27.811) knots 0 0 0 0 1 1 1 1
  spline S192 degree 3 poles (4.6654, 27.811) (4.3098, 27.0958) (4.1167, 26.7101) (4.0861, 26.6546) knots 0 0 0 0 1 1 1 1
  spline S193 degree 3 poles (4.0861, 26.6546) (4.056, 26.598) (4.0124, 26.5539) (3.9553, 26.5217) knots 0 0 0 0 1 1 1 1
  spline S194 degree 3 poles (3.9553, 26.5217) (3.8971, 26.49) (3.8369, 26.4739) (3.7746, 26.4739) knots 0 0 0 0 1 1 1 1
  spline S195 degree 3 poles (3.7746, 26.4739) (3.7139, 26.4739) (3.6553, 26.49) (3.5982, 26.5217) knots 0 0 0 0 1 1 1 1
  spline S196 degree 3 poles (3.5982, 26.5217) (3.5416, 26.5539) (3.4975, 26.598) (3.4653, 26.6546) knots 0 0 0 0 1 1 1 1
  spline S197 degree 3 poles (3.4653, 26.6546) (3.4336, 26.7101) (3.239, 27.0958) (2.8818, 27.811) knots 0 0 0 0 1 1 1 1
  spline S198 degree 3 poles (2.8818, 27.811) (2.5247, 28.5253) (2.3462, 28.9135) (2.3462, 28.9758) knots 0 0 0 0 1 1 1 1
  spline S199 degree 3 poles (2.3462, 28.9758) (2.3462, 29.0397) (2.3623, 29.0999) (2.3939, 29.1565) knots 0 0 0 0 1 1 1 1
  spline S200 degree 3 poles (2.3939, 29.1565) (2.4261, 29.2136) (2.4707, 29.2572) (2.5289, 29.2873) knots 0 0 0 0 1 1 1 1
  spline S201 degree 3 poles (2.5289, 29.2873) (2.586, 29.3179) (2.6441, 29.333) (2.7033, 29.333) knots 0 0 0 0 1 1 1 1
  line L87 (-6.6591, 9.4349) -> (-1.7809, 9.4349)
  spline S202 degree 3 poles (-1.7809, 9.4349) (-1.6424, 9.4349) (-1.509, 9.4008) (-1.3799, 9.3316) knots 0 0 0 0 1 1 1 1
  spline S203 degree 3 poles (-1.3799, 9.3316) (-1.2496, 9.2634) (-1.1483, 9.1642) (-1.0739, 9.0339) knots 0 0 0 0 1 1 1 1
  spline S204 degree 3 poles (-1.0739, 9.0339) (-1.0016, 8.9016) (-0.9664, 8.7642) (-0.9664, 8.6205) knots 0 0 0 0 1 1 1 1
  spline S205 degree 3 poles (-0.9664, 8.6205) (-0.9664, 8.48) (-1.3716, 7.5953) (-2.1819, 5.9664) knots 0 0 0 0 1 1 1 1
  spline S206 degree 3 poles (-2.1819, 5.9664) (-2.9942, 4.3355) (-3.4355, 3.4549) (-3.5048, 3.3247) knots 0 0 0 0 1 1 1 1
  spline S207 degree 3 poles (-3.5048, 3.3247) (-3.5761, 3.1955) (-3.6764, 3.0953) (-3.8066, 3.0229) knots 0 0 0 0 1 1 1 1
  spline S208 degree 3 poles (-3.8066, 3.0229) (-3.9358, 2.9516) (-4.0722, 2.9154) (-4.2159, 2.9154) knots 0 0 0 0 1 1 1 1
  spline S209 degree 3 poles (-4.2159, 2.9154) (-4.3564, 2.9154) (-4.4897, 2.9516) (-4.6169, 3.0229) knots 0 0 0 0 1 1 1 1
  spline S210 degree 3 poles (-4.6169, 3.0229) (-4.7461, 3.0953) (-4.8463, 3.1955) (-4.9187, 3.3247) knots 0 0 0 0 1 1 1 1
  spline S211 degree 3 poles (-4.9187, 3.3247) (-4.99, 3.4549) (-5.4334, 4.3355) (-6.2498, 5.9664) knots 0 0 0 0 1 1 1 1
  spline S212 degree 3 poles (-6.2498, 5.9664) (-7.0653, 7.5953) (-7.4735, 8.48) (-7.4735, 8.6205) knots 0 0 0 0 1 1 1 1
  spline S213 degree 3 poles (-7.4735, 8.6205) (-7.4735, 8.7642) (-7.4363, 8.9016) (-7.3619, 9.0339) knots 0 0 0 0 1 1 1 1
  spline S214 degree 3 poles (-7.3619, 9.0339) (-7.2896, 9.1642) (-7.1883, 9.2634) (-7.056, 9.3316) knots 0 0 0 0 1 1 1 1
  spline S215 degree 3 poles (-7.056, 9.3316) (-6.9258, 9.4008) (-6.7935, 9.4349) (-6.6591, 9.4349) knots 0 0 0 0 1 1 1 1
  spline S216 degree 3 poles (10.9056, 26.8352) (10.9045, 26.6001) (10.7851, 26.4796) (10.5484, 26.4739) knots 0 0 0 0 1 1 1 1
  line L88 (10.5484, 26.4739) -> (8.7421, 26.4781)
  spline S217 degree 3 poles (8.7421, 26.4781) (8.521, 26.4812) (8.4094, 26.5964) (8.4078, 26.8248) knots 0 0 0 0 1 1 1 1
  spline S218 degree 3 poles (8.4078, 26.8248) (8.4078, 27.0672) (8.5277, 27.1897) (8.767, 27.1923) knots 0 0 0 0 1 1 1 1
  line L89 (8.767, 27.1923) -> (10.1893, 27.1923)
  line L90 (10.1893, 27.1923) -> (10.1893, 28.6146)
  line L91 (10.1893, 28.6146) -> (8.7712, 28.6146)
  spline S219 degree 3 poles (8.7712, 28.6146) (8.5319, 28.6161) (8.412, 28.7365) (8.412, 28.9758) knots 0 0 0 0 1 1 1 1
  spline S220 degree 3 poles (8.412, 28.9758) (8.412, 29.2099) (8.5298, 29.3283) (8.7649, 29.3309) knots 0 0 0 0 1 1 1 1
  line L92 (8.7649, 29.3309) -> (10.5484, 29.3309)
  spline S221 degree 3 poles (10.5484, 29.3309) (10.7851, 29.3309) (10.9045, 29.2156) (10.9056, 28.9841) knots 0 0 0 0 1 1 1 1
  line L93 (10.9056, 28.9841) -> (10.9056, 26.8352)
  spline S222 degree 3 poles (24.8226, 26.8352) (24.8226, 26.6001) (24.7038, 26.4812) (24.4655, 26.4781) knots 0 0 0 0 1 1 1 1
  line L94 (24.4655, 26.4781) -> (23.2177, 26.4781)
  spline S223 degree 3 poles (23.2177, 26.4781) (22.981, 26.4781) (22.7728, 26.5674) (22.5927, 26.7459) knots 0 0 0 0 1 1 1 1
  spline S224 degree 3 poles (22.5927, 26.7459) (22.4116, 26.9245) (22.3223, 27.1332) (22.3249, 27.3709) knots 0 0 0 0 1 1 1 1
  spline S225 degree 3 poles (22.3249, 27.3709) (22.328, 27.6091) (22.3892, 27.7856) (22.5097, 27.9003) knots 0 0 0 0 1 1 1 1
  spline S226 degree 3 poles (22.5097, 27.9003) (22.3841, 28.0239) (22.3223, 28.2029) (22.3249, 28.4381) knots 0 0 0 0 1 1 1 1
  spline S227 degree 3 poles (22.3249, 28.4381) (22.3264, 28.6737) (22.4162, 28.8814) (22.5948, 29.061) knots 0 0 0 0 1 1 1 1
  spline S228 degree 3 poles (22.5948, 29.061) (22.7734, 29.2411) (22.9737, 29.3309) (23.1948, 29.3309) knots 0 0 0 0 1 1 1 1
  line L95 (23.1948, 29.3309) -> (24.4697, 29.3309)
  spline S229 degree 3 poles (24.4697, 29.3309) (24.7053, 29.3335) (24.8226, 29.2146) (24.8226, 28.9738) knots 0 0 0 0 1 1 1 1
  line L96 (24.8226, 28.9738) -> (24.8226, 26.8352)
sketch "Sketch7" plane through (0, 0, 2) normal (0, 0, 1) x (1, 0, 0)
